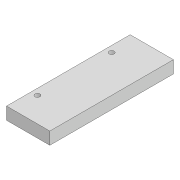
# Autodesk Inventor part: Крепление для опор
Saved by Autodesk Inventor 2022 (Build 260153000, 153)
## iProperties
Created: 2023-02-20
Part Number: Крепление для опор
Material: Типовые
Document SubType Name: Modeling
Designer: Глеб
Density: 1 g/cm^3
Appearance: По умолчанию
Author: Глеб
Autodesk Inventor part; units mm, degrees
ref_plane "YZ Plane" through (0, 0, 0) normal (1, 0, 0) x (0, 1, 0)
ref_plane "XZ Plane" through (0, 0, 0) normal (0, 1, 0) x (-1, 0, 0)
ref_plane "XY Plane" through (0, 0, 0) normal (0, 0, 1) x (1, 0, 0)
sketch "Эскиз1" plane through (0, 0, 0) normal (0, 1, 0) x (-1, 0, 0)
  line L0 (-35, 90) -> (35, 90)
  line L1 (35, 90) -> (35, -90)
  line L2 (35, -90) -> (-35, -90)
  line L3 (-35, -90) -> (-35, 90)
  line L4 (-35, 90) -> (35, -90) construction
  line L5 (35, 90) -> (-35, -90) construction
  point P0 (0, 0)
  dimension "d0" = 70
  dimension "d1" = 180
  constraints: 12 end point, 2 midpoint, 2 parallel, 1 horizontal, 1 perpendicular
  measures "d0" distance of L1.end L2.end
  measures "d1" distance of L0.end L1.end
extrude "Выдавливание1" add sketch "Эскиз1" along normal blind 20
sketch "Эскиз2" plane through (0, 20, 0) normal (0, 1, 0) x (1, 0, 0)
  line L0 (-38.8888, 0) -> (-2.6205, 0) construction
  line L1 (-35, 90) -> (-35, -90) projected
  point P0 (0, 0)
  point P1 (-29, -60)
  point P2 (-29, 60)
  dimension "d5" = 60
  dimension "d13" = 6
  constraints: 2 end point, 1 horizontal, 1 symmetric about line
  measures "d5" distance from line of point (-29, -60) L0
  measures "d13" distance from line of L1 point (-29, -60)
hole "Отверстие1" at (-29, 20, 60) at (-29, 20, -60) direction (0, -1, 0) diameter 8.1 depth 80
